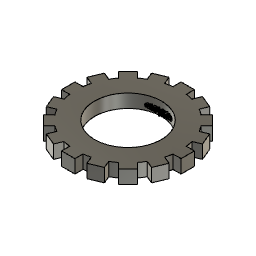
Model 14 (Autodesk Fusion 360 design; units mm, degrees)
Autodesk Fusion 360 part; units mm, degrees
sketch "Sketch2" plane through (0, 0, 0) normal (0, 0, 1) x (1, 0, 0)
  circle A0 centre (0, 0) radius 25
  circle A1 centre (0, 0) radius 39
  line L0 (0, 0) -> (0, 45) construction
  line L1 (0, 0) -> (45, 0) construction
  line L2 (0, 0) -> (-45, 0) construction
  line L3 (0, 0) -> (0, -45) construction
  line L4 (5, 38.6782) -> (5, 44.7214)
  line L5 (5, 44.7214) -> (0, 44.7214)
  line L6 (0, 44.7214) -> (-5, 44.7214)
  line L7 (-5, 38.6782) -> (-5, 44.7214)
  arc A2 (-5, 44.7214) -> (5, 44.7214) centre (0, 0) ccw construction
  line L8 (-19.4209, 33.8205) -> (-21.7335, 39.4037)
  line L9 (-17.1141, 41.3171) -> (-21.7335, 39.4037)
  line L10 (-12.4947, 43.2306) -> (-17.1141, 41.3171)
  line L11 (-10.1821, 37.6474) -> (-12.4947, 43.2306)
  line L12 (-30.8851, 23.8141) -> (-35.1583, 28.0872)
  line L13 (-31.6228, 31.6228) -> (-35.1583, 28.0872)
  line L14 (-28.0872, 35.1583) -> (-31.6228, 31.6228)
  line L15 (-23.8141, 30.8851) -> (-28.0872, 35.1583)
  line L16 (-37.6474, 10.1821) -> (-43.2306, 12.4947)
  line L17 (-41.3171, 17.1141) -> (-43.2306, 12.4947)
  line L18 (-39.4037, 21.7335) -> (-41.3171, 17.1141)
  line L19 (-33.8205, 19.4209) -> (-39.4037, 21.7335)
  line L20 (-38.6782, -5) -> (-44.7214, -5)
  line L21 (-44.7214, 0) -> (-44.7214, -5)
  line L22 (-44.7214, 5) -> (-44.7214, 0)
  line L23 (-38.6782, 5) -> (-44.7214, 5)
  line L24 (-33.8205, -19.4209) -> (-39.4037, -21.7335)
  line L25 (-41.3171, -17.1141) -> (-39.4037, -21.7335)
  line L26 (-43.2306, -12.4947) -> (-41.3171, -17.1141)
  line L27 (-37.6474, -10.1821) -> (-43.2306, -12.4947)
  line L28 (-23.8141, -30.8851) -> (-28.0872, -35.1583)
  line L29 (-31.6228, -31.6228) -> (-28.0872, -35.1583)
  line L30 (-35.1583, -28.0872) -> (-31.6228, -31.6228)
  line L31 (-30.8851, -23.8141) -> (-35.1583, -28.0872)
  line L32 (-10.1821, -37.6474) -> (-12.4947, -43.2306)
  line L33 (-17.1141, -41.3171) -> (-12.4947, -43.2306)
  line L34 (-21.7335, -39.4037) -> (-17.1141, -41.3171)
  line L35 (-19.4209, -33.8205) -> (-21.7335, -39.4037)
  line L36 (5, -38.6782) -> (5, -44.7214)
  line L37 (0, -44.7214) -> (5, -44.7214)
  line L38 (-5, -44.7214) -> (0, -44.7214)
  line L39 (-5, -38.6782) -> (-5, -44.7214)
  line L40 (19.4209, -33.8205) -> (21.7335, -39.4037)
  line L41 (17.1141, -41.3171) -> (21.7335, -39.4037)
  line L42 (12.4947, -43.2306) -> (17.1141, -41.3171)
  line L43 (10.1821, -37.6474) -> (12.4947, -43.2306)
  line L44 (30.8851, -23.8141) -> (35.1583, -28.0872)
  line L45 (31.6228, -31.6228) -> (35.1583, -28.0872)
  line L46 (28.0872, -35.1583) -> (31.6228, -31.6228)
  line L47 (23.8141, -30.8851) -> (28.0872, -35.1583)
  line L48 (37.6474, -10.1821) -> (43.2306, -12.4947)
  line L49 (41.3171, -17.1141) -> (43.2306, -12.4947)
  line L50 (39.4037, -21.7335) -> (41.3171, -17.1141)
  line L51 (33.8205, -19.4209) -> (39.4037, -21.7335)
  line L52 (38.6782, 5) -> (44.7214, 5)
  line L53 (44.7214, 0) -> (44.7214, 5)
  line L54 (44.7214, -5) -> (44.7214, 0)
  line L55 (38.6782, -5) -> (44.7214, -5)
  line L56 (33.8205, 19.4209) -> (39.4037, 21.7335)
  line L57 (41.3171, 17.1141) -> (39.4037, 21.7335)
  line L58 (43.2306, 12.4947) -> (41.3171, 17.1141)
  line L59 (37.6474, 10.1821) -> (43.2306, 12.4947)
  line L60 (23.8141, 30.8851) -> (28.0872, 35.1583)
  line L61 (31.6228, 31.6228) -> (28.0872, 35.1583)
  line L62 (35.1583, 28.0872) -> (31.6228, 31.6228)
  line L63 (30.8851, 23.8141) -> (35.1583, 28.0872)
  line L64 (10.1821, 37.6474) -> (12.4947, 43.2306)
  line L65 (17.1141, 41.3171) -> (12.4947, 43.2306)
  line L66 (21.7335, 39.4037) -> (17.1141, 41.3171)
  line L67 (19.4209, 33.8205) -> (21.7335, 39.4037)
  dimension "d26" = 50
  dimension "d27" = 78
  dimension "d28" = 90
  dimension "d32" = 360
  constraint coincident A0.centre A1.centre
  constraint concentric A0 A1
  constraint concentric A1 A2
  constraint vertical L0
  constraint coincident L1.end A2
  constraint perpendicular L0 L1
  constraint coincident L2.end A2
  constraint parallel L1 L2
  constraint coincident L3.end A2
  constraint perpendicular L2 L3
  constraint coincident L0 L5.end
  constraint perpendicular L0 L5
  constraint perpendicular L0 L6
  constraint coincident A1 L7.start
  constraint coincident A1 L4.start
  measures "d26" diameter of A0
  measures "d27" diameter of A1
  measures "d28" diameter of A2
extrude "Extrude2" add sketch "Sketch2" along normal blind 10
ref_plane "WorkPlane1" through (0, 25, 3.8908) normal (0, -1, 0) x (-1, 0, 0)
ref_plane "WorkPlane2" through (0, 22, 3.8908) normal (0, -1, 0) x (-1, 0, 0)
sketch "Sketch3" plane through (0, 25, 3.8908) normal (0, -1, 0) x (1, 0, 0)
  line L0 (-14.3191, -2.2363) -> (14.6839, -1.9476) construction
  line L1 (14.6839, -1.9476) -> (14.6403, 2.4295) construction
  line L2 (14.6403, 2.4295) -> (-14.3626, 2.1408) construction
  line L3 (-14.3626, 2.1408) -> (-14.3191, -2.2363) construction
  text T0 "enes şahin" font "Arial" height 3 align centre top in box 29.0044 x 4.3774 at (-14.3191, -2.2363) x (0.99995, 0.009955) y (-0.009955, 0.99995) spacing 1
extrude "Extrude3" add sketch "Sketch3" along normal blind 3 text T0
